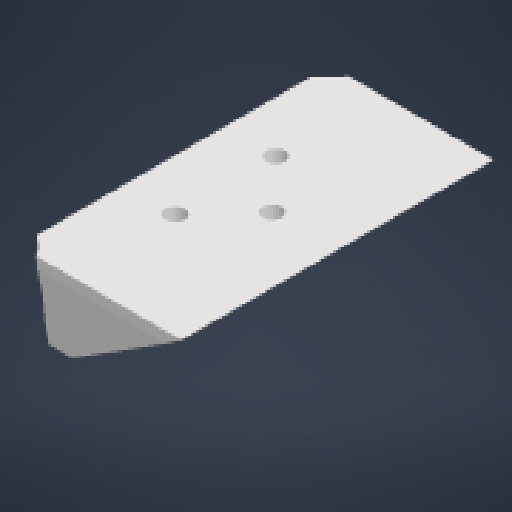
# Autodesk Inventor part: Head_Fin_Bottom
Saved by Autodesk Inventor 2024 (Build 280153000, 153)
## iProperties
Created: 2025-09-26
Part Number: Head_Fin_Bottom
Material: Generic
Document SubType Name: Modeling
Designer: kevin
Density: 1 g/cm^3
Appearance: Default
Author: kevin
Autodesk Inventor part; units mm, degrees
ref_plane "YZ Plane" through (0, 0, 0) normal (1, 0, 0) x (0, 1, 0)
ref_plane "XZ Plane" through (0, 0, 0) normal (0, 1, 0) x (-1, 0, 0)
ref_plane "XY Plane" through (0, 0, 0) normal (0, 0, 1) x (1, 0, 0)
sketch "Sketch1" plane through (0, 0, 0) normal (0, 0, 1) x (1, 0, 0)
  line L0 (-108.119909, -0.642406) -> (-283.474909, -0.642406)
  line L1 (-142.122291, -0.642406) -> (-170.837871, -20.749272)
  line L2 (-142.122291, -0.642406) -> (-107.067041, -0.642406) construction
  line L3 (-170.837871, -20.749272) -> (-177.837871, -20.749272)
  line L4 (-177.837871, -20.749272) -> (-184.577322, -0.642406)
  line L5 (-177.837871, -20.749272) -> (-177.837871, -0.642406)
  point P0 (0, 0)
  dimension "d0" = 145
  dimension "d1" = 7
  constraints: 10 end point, 3 point on line, 2 horizontal, 1 equal length, 1 perpendicular
  measures "d0" angle of L1 L2
  measures "d1" distance of L1.end L3.end
extrude "Extrusion1" add sketch "Sketch1" along normal mid plane 68.2625 contours L1 L3 L5 L0
chamfer "Chamfer1" distance 4.7625 angle 75 2 edges at (-174.3379, -20.7493, -34.1313) (-174.3379, -20.7493, 34.1313) measured on face at (-175.5045, -20.7493, -11.3771)
chamfer "Chamfer2" distance 2 angle 45 1 edges at (-177.8379, -20.7493, 0)
sketch "Sketch2" plane through (-177.837871, -0.642406, 34.13125) normal (0, 1, 0) x (1, 0, 0)
  circle A0 centre (11.158205, 23.13125) radius 2.1
  circle A1 centre (21.356244, 34.13125) radius 2.1
  circle A2 centre (11.158205, 45.13125) radius 2.1
  point P0 (177.837871, 34.13125)
extrude "Extrusion2" cut sketch "Sketch2" against normal blind 5.5
sketch "Sketch3" plane through (-177.837871, -0.642406, 34.13125) normal (0, 1, 0) x (1, 0, 0)
  ellipse E0 centre (-9.038126, 75.297581) end of major axis (-3.616987, 62.831943) minor radius 11.723829
  ellipse E1 centre (-5.030683, 77.040364) end of major axis (-0.216713, 65.970883) minor radius 10.410756
  ellipse E2 centre (-9.038126, 75.297581) end of major axis (-3.616987, 62.831943) minor radius 11.723829
  ellipse E3 centre (-5.030683, 77.040364) end of major axis (-0.216713, 65.970883) minor radius 10.410756
  circle A0 centre (-7.965707, 75.900412) radius 14.145392
  line L0 (35.71558, 68.2625) -> (35.71558, 0)
  line L1 (35.71558, 34.13125) -> (24.180949, 34.13125) construction
  circle A1 centre (-7.965707, -7.637912) radius 14.145392
  point P0 (177.837871, 34.13125)
  constraints: 2 centre point, 2 end point, 1 horizontal, 1 midpoint, 1 symmetric about line, 1 other
sketch "Sketch3 outline for Extrusion3" plane through (-177.837871, -0.642406, 34.13125) normal (0, 1, 0) x (1, 0, 0)
  circle A0 centre (-7.965707, -7.637912) radius 14.145392
  circle A1 centre (-7.965707, 75.900412) radius 14.145392
extrude "Extrusion3" cut sketch "Sketch3 outline for Extrusion3" against normal blind 25.4 draft 5
body "Solid1"
